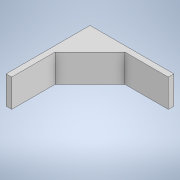
# Autodesk Inventor part: уголок
Saved by Autodesk Inventor 2021.1 (Build 251245010, 245A)
## iProperties
Created: 2021-07-16
Part Number: уголок
Material: Типовые
Document SubType Name: Modeling
Designer: User
Density: 1 g/cm^3
Appearance: По умолчанию
Author: User
Autodesk Inventor part; units mm, degrees
ref_plane "YZ Plane" through (0, 0, 0) normal (1, 0, 0) x (0, 1, 0)
ref_plane "XZ Plane" through (0, 0, 0) normal (0, 1, 0) x (-1, 0, 0)
ref_plane "XY Plane" through (0, 0, 0) normal (0, 0, 1) x (1, 0, 0)
sketch "Эскиз1" plane through (0, 0, 0) normal (0, 1, 0) x (-1, 0, 0)
  line L0 (0, 0) -> (-4, 0)
  line L1 (-4, 29) -> (-4, 60)
  line L2 (-4, 60) -> (0, 60)
  line L3 (0, 60) -> (0, 0)
  line L4 (0, 0) -> (-60, 0)
  line L5 (-60, 0) -> (-60, 4)
  line L6 (-60, 4) -> (-29, 4)
  line L7 (0, 4) -> (0, 0)
  line L8 (-4, 29) -> (-29, 4)
  dimension "d0" = 4
  dimension "d1" = 60
  dimension "d2" = 60
  dimension "d3" = 4
  dimension "d4" = 25
  dimension "d5" = 25
  constraints: 18 end point, 4 parallel, 2 horizontal, 2 perpendicular
  measures "d0" distance of L1.end L2.end
  measures "d1" distance of L0.end L1.end
  measures "d2" distance of L5.end L7.start
  measures "d3" distance of L4.end L5.end
  measures "d4" distance from line of L1.start L6
  measures "d5" distance from line of L6.end L1
extrude "Выдавливание1" add sketch "Эскиз1" along normal blind 20
